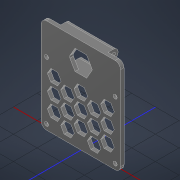
# Autodesk Inventor part: Base-Plate
Saved by Autodesk Inventor 2022.2 (Build 262287010, 287A)
## iProperties
Created: 2022-03-22
Part Number: Base-Plate
Material: ABS-Kunststoff
Document SubType Name: Modeling
Designer: sleib
Density: 1.06 g/cm^3
Appearance: Glatt - Schwarz
Author: sleib
Autodesk Inventor part; units mm, degrees
ref_plane "YZ Plane" through (0, 0, 0) normal (1, 0, 0) x (0, 1, 0)
ref_plane "XZ Plane" through (0, 0, 0) normal (0, 1, 0) x (-1, 0, 0)
ref_plane "XY Plane" through (0, 0, 0) normal (0, 0, 1) x (1, 0, 0)
sketch "Skizze1" plane through (0, 0, 0) normal (1, 0, 0) x (0, 1, 0)
  line L0 (33, 3) -> (-47, 3)
  line L1 (-47, 3) -> (-47, 0)
  line L2 (-47, 0) -> (33, 0)
  line L3 (33, 0) -> (33, 3)
  line L4 (33, 0) -> (25, 0)
  line L5 (25, 0) -> (25, -4.5)
  line L6 (25, -4.5) -> (33, -4.5) construction
  line L7 (33, -4.5) -> (33, 0)
  circle A0 centre (29, -4.5) radius 4
  line L8 (8, 0) -> (0, 0)
  line L9 (0, 0) -> (0, -8.5)
  line L10 (0, -8.5) -> (8, -8.5) construction
  line L11 (8, -8.5) -> (8, 0)
  circle A1 centre (4, -8.5) radius 4
  circle A2 centre (29, -4.5) radius 1.7
  circle A3 centre (4, -8.5) radius 1.7
  dimension "d0" = 80
  dimension "d1" = 3
  dimension "d2" = 8
  dimension "d5" = 4.5
  dimension "d6" = 8
  dimension "d7" = 8.5
  dimension "d8" = 25
  dimension "d9" = 3.4
  dimension "d10" = 3.4
  constraints: 24 end point, 6 parallel, 3 coincident, 3 horizontal, 3 perpendicular, 2 centre point, 2 midpoint, 1 point on line, 6 other
  measures "d0" distance between parallel lines of L1 L3
  measures "d1" distance of L2.end L0.start
  measures "d2" distance of L6.end L5.end
  measures "d5" distance between parallel lines of L4 L6
  measures "d6" distance of L10.end L9.end
  measures "d7" distance between parallel lines of L10 L8
  measures "d8" horizontal distance of point (4, -8.5) point (29, -4.5)
  measures "d9" diameter of A2
  measures "d10" diameter of A3
extrude "Extrusion1" add sketch "Skizze1" along normal mid plane 67 contours L3 L2 L1 L0
extrude "Extrusion2" add sketch "Skizze1" along normal mid plane 40 contours L7 A0 L5 L2 | A0
extrude "Extrusion3" add sketch "Skizze1" along normal mid plane 26 contours L2 L11 A1 L9 | A1
sketch "Skizze3" plane through (33.5, -47, 0) normal (0, 0, -1) x (-1, 0, 0)
  line L0 (13.5, 72) -> (13.5, 80) projected
  line L1 (13.5, 80) -> (0, 80) projected
  line L2 (0, 0) -> (0, 80) projected
  line L3 (0, 0) -> (67, 0) projected
  line L4 (67, 80) -> (67, 0) projected
  line L5 (67, 80) -> (53.5, 80) projected
  line L6 (53.5, 80) -> (53.5, 72) projected
  line L7 (53.5, 72) -> (13.5, 72) projected
  circle A0 centre (4.5, 4.5) radius 4.5 construction
  circle A1 centre (62.5, 4.5) radius 4.5 construction
  line L8 (0, 0) -> (0, 80) projected
  line L9 (67, 80) -> (67, 0) projected
  line L10 (0, 0) -> (67, 0) projected
  circle A2 centre (4.5, 4.5) radius 1.7
  circle A3 centre (62.5, 4.5) radius 1.7
  circle A4 centre (4.5, 53.5) radius 1.7
  circle A5 centre (62.5, 53.5) radius 1.7
  line L11 (67, 80) -> (0, 80) construction
  line L12 (33.5, 80) -> (33.5, 0) construction
  line L13 (67, 0) -> (0, 0) construction
  line L14 (38.4075, 55) -> (28.5925, 55)
  line L15 (28.5925, 55) -> (23.685, 63.5)
  line L16 (23.685, 63.5) -> (28.5925, 72)
  line L17 (28.5925, 72) -> (38.4075, 72)
  line L18 (38.4075, 72) -> (43.315, 63.5)
  line L19 (43.315, 63.5) -> (38.4075, 55)
  line L20 (53.5, 72) -> (13.5, 72) projected
  circle A6 centre (4.5, 4.5) radius 3
  circle A7 centre (62.5, 4.5) radius 3
  circle A8 centre (62.5, 53.5) radius 3
  circle A9 centre (4.5, 53.5) radius 3
  line L21 (13.8701, 37) -> (8.0966, 37)
  line L22 (8.0966, 37) -> (5.2098, 42)
  line L23 (5.2098, 42) -> (8.0966, 47)
  line L24 (8.0966, 47) -> (13.8701, 47)
  line L25 (13.8701, 47) -> (16.7568, 42)
  line L26 (16.7568, 42) -> (13.8701, 37)
  line L27 (25.1284, 30.5) -> (19.3549, 30.5)
  line L28 (19.3549, 30.5) -> (16.4682, 35.5)
  line L29 (16.4682, 35.5) -> (19.3549, 40.5)
  line L30 (19.3549, 40.5) -> (25.1284, 40.5)
  line L31 (25.1284, 40.5) -> (28.0152, 35.5)
  line L32 (28.0152, 35.5) -> (25.1284, 30.5)
  line L33 (80.4, 47) -> (-13.4, 47) construction
  line L34 (33.5, -19.1324) -> (33.5, 96.5221) construction
  line L35 (30.6132, 37) -> (27.7265, 42)
  line L36 (27.7265, 42) -> (30.6132, 47)
  line L37 (30.6132, 47) -> (36.3868, 47)
  line L38 (36.3868, 37) -> (30.6132, 37)
  line L39 (36.3868, 47) -> (39.2735, 42)
  line L40 (39.2735, 42) -> (36.3868, 37)
  line L41 (53.1299, 37) -> (50.2432, 42)
  line L42 (50.2432, 42) -> (53.1299, 47)
  line L43 (53.1299, 47) -> (58.9034, 47)
  line L44 (58.9034, 37) -> (53.1299, 37)
  line L45 (58.9034, 47) -> (61.7902, 42)
  line L46 (61.7902, 42) -> (58.9034, 37)
  line L47 (8.0966, 24) -> (5.2098, 29)
  line L48 (5.2098, 29) -> (8.0966, 34)
  line L49 (8.0966, 34) -> (13.8701, 34)
  line L50 (13.8701, 24) -> (8.0966, 24)
  line L51 (13.8701, 34) -> (16.7568, 29)
  line L52 (16.7568, 29) -> (13.8701, 24)
  line L53 (30.6132, 24) -> (27.7265, 29)
  line L54 (27.7265, 29) -> (30.6132, 34)
  line L55 (30.6132, 34) -> (36.3868, 34)
  line L56 (36.3868, 24) -> (30.6132, 24)
  line L57 (36.3868, 34) -> (39.2735, 29)
  line L58 (39.2735, 29) -> (36.3868, 24)
  line L59 (53.1299, 24) -> (50.2432, 29)
  line L60 (50.2432, 29) -> (53.1299, 34)
  line L61 (53.1299, 34) -> (58.9034, 34)
  line L62 (58.9034, 24) -> (53.1299, 24)
  line L63 (58.9034, 34) -> (61.7902, 29)
  line L64 (61.7902, 29) -> (58.9034, 24)
  line L65 (8.0966, 11) -> (5.2098, 16)
  line L66 (5.2098, 16) -> (8.0966, 21)
  line L67 (8.0966, 21) -> (13.8701, 21)
  line L68 (13.8701, 11) -> (8.0966, 11)
  line L69 (13.8701, 21) -> (16.7568, 16)
  line L70 (16.7568, 16) -> (13.8701, 11)
  line L71 (30.6132, 11) -> (27.7265, 16)
  line L72 (27.7265, 16) -> (30.6132, 21)
  line L73 (30.6132, 21) -> (36.3868, 21)
  line L74 (36.3868, 11) -> (30.6132, 11)
  line L75 (36.3868, 21) -> (39.2735, 16)
  line L76 (39.2735, 16) -> (36.3868, 11)
  line L77 (53.1299, 11) -> (50.2432, 16)
  line L78 (50.2432, 16) -> (53.1299, 21)
  line L79 (53.1299, 21) -> (58.9034, 21)
  line L80 (58.9034, 11) -> (53.1299, 11)
  line L81 (58.9034, 21) -> (61.7902, 16)
  line L82 (61.7902, 16) -> (58.9034, 11)
  line L83 (38.9848, 35.5) -> (41.8716, 40.5)
  line L84 (41.8716, 30.5) -> (38.9848, 35.5)
  line L85 (41.8716, 40.5) -> (47.6451, 40.5)
  line L86 (47.6451, 30.5) -> (41.8716, 30.5)
  line L87 (47.6451, 40.5) -> (50.5318, 35.5)
  line L88 (50.5318, 35.5) -> (47.6451, 30.5)
  line L89 (16.4682, 22.5) -> (19.3549, 27.5)
  line L90 (19.3549, 17.5) -> (16.4682, 22.5)
  line L91 (19.3549, 27.5) -> (25.1284, 27.5)
  line L92 (25.1284, 17.5) -> (19.3549, 17.5)
  line L93 (25.1284, 27.5) -> (28.0152, 22.5)
  line L94 (28.0152, 22.5) -> (25.1284, 17.5)
  line L95 (38.9848, 22.5) -> (41.8716, 27.5)
  line L96 (41.8716, 17.5) -> (38.9848, 22.5)
  line L97 (41.8716, 27.5) -> (47.6451, 27.5)
  line L98 (47.6451, 17.5) -> (41.8716, 17.5)
  line L99 (47.6451, 27.5) -> (50.5318, 22.5)
  line L100 (50.5318, 22.5) -> (47.6451, 17.5)
  line L101 (16.4682, 9.5) -> (19.3549, 14.5)
  line L102 (19.3549, 4.5) -> (16.4682, 9.5)
  line L103 (19.3549, 14.5) -> (25.1284, 14.5)
  line L104 (25.1284, 4.5) -> (19.3549, 4.5)
  line L105 (25.1284, 14.5) -> (28.0152, 9.5)
  line L106 (28.0152, 9.5) -> (25.1284, 4.5)
  line L107 (38.9848, 9.5) -> (41.8716, 14.5)
  line L108 (41.8716, 4.5) -> (38.9848, 9.5)
  line L109 (41.8716, 14.5) -> (47.6451, 14.5)
  line L110 (47.6451, 4.5) -> (41.8716, 4.5)
  line L111 (47.6451, 14.5) -> (50.5318, 9.5)
  line L112 (50.5318, 9.5) -> (47.6451, 4.5)
  line L113 (46.5, 55) -> (20.5, 55) projected
  line L114 (20.5, 47) -> (20.5, 55) projected
  line L115 (46.5, 47) -> (20.5, 47) projected
  line L116 (46.5, 55) -> (46.5, 47) projected
  point P0 (33.5, 47)
  point P1 (33.5, 63.5)
  point P2 (10.9833, 42)
  point P3 (22.2417, 35.5)
  point P4 (33.5, 42)
  point P5 (56.0167, 42)
  point P6 (10.9833, 29)
  point P7 (33.5, 29)
  point P8 (56.0167, 29)
  point P9 (10.9833, 16)
  point P10 (33.5, 16)
  point P11 (56.0167, 16)
  point P12 (44.7583, 35.5)
  point P13 (22.2417, 22.5)
  point P14 (44.7583, 22.5)
  point P15 (22.2417, 9.5)
  point P16 (44.7583, 9.5)
  dimension "d19" = 9
  dimension "d20" = 3.4
  dimension "d21" = 49
  dimension "d25" = 6
  dimension "d28" = 10
  dimension "d29" = 10
  dimension "d30" = 3
  dimension "d31" = 1.5
  dimension "d32" = 11.2583
  dimension "d35" = 22.5167
  dimension "d38" = 13
  dimension "d43" = 22.5167
  dimension "d46" = 13
  constraints: 194 end point, 10 centre point, 7 equal radius, 6 coincident, 4 horizontal, 4 tangent, 3 collinear, 2 midpoint, 2 point on line, 2 vertical, 2 vertical alignment, 1 horizontal alignment, 208 other
  measures "d19" diameter of A0
  measures "d20" diameter of A2
  measures "d21" distance of A2.centre A4.centre
  measures "d25" diameter of A6
  measures "d28" distance between parallel lines of L21 L24
  measures "d29" distance between parallel lines of L27 L30
  measures "d30" distance between parallel lines of L29 L26
  measures "d31" distance from line of L30 L25.end
  measures "d32" horizontal distance of point (22.242, 35.5) point (10.983, 42)
  measures "d35" distance of L22.end L35.end
  measures "d38" distance of L22.end L47.end
  measures "d43" distance of L29.end L83.end
  measures "d46" distance of L29.end L89.end
extrude "Extrusion4" cut sketch "Skizze3" against normal through all contours L7 L18 L19 L14 L15 L16 | L37 L39 L40 L38 L35 L36 | A2 | A3 | A4 | A5 | L21 L22 L23 L24 L25 L26 | L27 L28 L29 L30 L31 L32 | L41 L42 L43 L45 L46 L44 | L47 L48 L49 L51 L52 L50 | L53 L54 L55 L57 L58 L56 | L59 L60 L61 L63 L64 L62 | L65 L66 L67 L69 L70 L68 | L71 L72 L73 L75 L76 L74 | L77 L78 L79 L81 L82 L80 | L83 L85 L87 L88 L86 L84 | L89 L91 L93 L94 L92 L90 | L95 L97 L99 L100 L98 L96 | L101 L103 L105 L106 L104 L102 | L107 L109 L111 L112 L110 L108
extrude "Extrusion5" cut sketch "Skizze3" against normal blind 1 contours A6 | A7 | A8 | A9
fillet "Rundung1" radius 4.5 4 edges at (33.5, -47, 1.5) (-33.5, -47, 1.5) (-33.5, 33, 1.5) (33.5, 33, 1.5)
fillet "Rundung2" radius 2 2 edges at (-9.815, 16.5, 1.5) (9.815, 16.5, 1.5)
equation "\"d29\" = d28"
equation "\"d31\" = 0.5 * d30"
equation "\"d35\" = 2 * d32"
equation "\"d38\" = d28 + d30"
equation "\"d43\" = 2 * d32"
equation "\"d46\" = d28 + d30"
